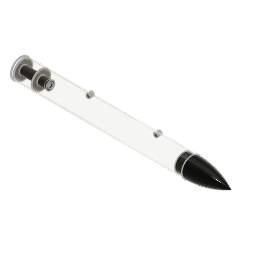
Alpha v1 v2 (Autodesk Fusion 360 design; units mm, degrees)
Autodesk Fusion 360 part; units mm, degrees
sketch "Fuselage" plane through (0, 0, 0) normal (1, 0, 0) x (0, 1, 0)
  circle A0 centre (0, 0) radius 25
  dimension "d1" = 50
  constraint coincident A0.centre origin
  measures "d1" diameter of A0
extrude "Extrude1" add sketch "Fuselage" along normal blind 430 thin wall 2 inside makes body 1
sketch "Ogive" plane through (430, 0, 0) normal (1, 0, 0) x (0, 1, 0)
  circle A0 centre (0, 0) radius 23
  circle A1 centre (0, 0) radius 25
  circle A2 centre (0, 0) radius 25
  line L0 (0, 25) -> (0, -25)
  constraint concentric A0 A2
  constraint coincident A2 L0.start
  constraint coincident A2 L0.end
  constraint vertical L0
extrude "Extrude2" add sketch "Ogive" along normal blind 100 separate body contours A0 L0 | A0 A1 A2 L0 picked at (5.0206, 5.7941) picked at (1.186, 24.2485) makes body 2
sketch "Ogive Curvature Profile" plane through (0, 0, 0) normal (0, -1, 0) x (1, 0, 0)
  line L0 (430, 25) -> (430, -25)
  line L1 (430, -25) -> (530, -25)
  line L2 (530, -25) -> (530, 25)
  line L3 (530, 25) -> (430, 25)
  line L4 (430, 0) -> (430, 25)
  line L5 (430, 0) -> (530, 0)
  circle A0 centre (430, -187.5) radius 212.5
  dimension "d7" = 212.5
  constraint midpoint L0 L4.start
  constraint coincident L0.start L3.end
  constraint midpoint L2 L5.end
  constraint coincident L0.start A0
  measures "d7" distance of L0.start A0.centre
extrude "Extrude3" add sketch "Ogive" along normal blind 100 contours A0 L0 | A0 A1 A2 L0 picked at (-4.3188, 6.3345) picked at (-2.3847, 24.1546) bodies 2
revolve "Revolve1" cut sketch "Ogive Curvature Profile" angle 360 about axis through (430, 0, 0) along (1, 0, 0) contours L0 L4 L5 A0 keep common part bodies 2
sketch "Sholder" plane through (430, 0, 0) normal (-1, 0, 0) x (0, -1, 0)
  circle A0 centre (0, 0) radius 25
  circle A1 centre (0, 0) radius 22.5
  dimension "d11" = 45
  constraint coincident A0.centre A1.centre
  measures "d11" diameter of A1
extrude "Extrude4" add sketch "Sholder" along normal blind 20 contours A1 bodies 2
sketch "Sholder Dent" plane through (410, 0, 0) normal (-1, 0, 0) x (0, -1, 0)
  circle A0 centre (0, 0) radius 22.5
  circle A1 centre (0, 0) radius 17.5
  line L0 (3.75, 17.5) -> (-3.75, 17.5)
  line L1 (-3.75, 17.5) -> (-3.75, -17.5)
  line L2 (-3.75, -17.5) -> (3.75, -17.5)
  line L3 (3.75, -17.5) -> (3.75, 17.5)
  line L4 (3.75, 17.5) -> (-3.75, -17.5) construction
  line L5 (-3.75, 17.5) -> (3.75, -17.5) construction
  dimension "d21" = 35
  dimension "d22" = 7.5
  dimension "d23" = 35
  constraint coincident A0.centre A1.centre
  constraint horizontal L0
  constraint perpendicular L0 L1
  constraint parallel L0 L2
  constraint parallel L1 L3
  constraint coincident L4 A0.centre
  constraint coincident L5 A0.centre
  measures "d21" diameter of A1
  measures "d22" distance of L1.end L2.end
  measures "d23" distance of L0.end L1.end
extrude "Extrude5" cut sketch "Sholder Dent" against normal blind 20 contours A1 L3 | A1 L1 bodies 2
sketch "Sholder Shock Cord hole" plane through (0, 3.75, 0) normal (0, 1, 0) x (-1, 0, 0)
  line L0 (-410, -17.0935) -> (-410, 17.0935)
  line L1 (-410, 17.0935) -> (-430, 17.0935)
  line L2 (-430, 17.0935) -> (-430, -17.0935)
  line L3 (-430, -17.0935) -> (-410, -17.0935)
  circle A0 centre (-420, 0) radius 5
  dimension "d29" = 10
  measures "d29" diameter of A0
extrude "Extrude7" cut sketch "Sholder Shock Cord hole" against normal blind 7.5 contours A0 bodies 2
sketch "Rail Button" plane through (0, 0, 0) normal (0, 0, 1) x (1, 0, 0)
  line L0 (0, 0) -> (5, 0)
  line L1 (0, 0) -> (0, 2)
  line L2 (5, 0) -> (5, 5)
  line L3 (5, 5) -> (1, 5)
  line L4 (1, 5) -> (1, 2)
  line L5 (0, 2) -> (2.1888, 2)
  line L6 (1, 5) -> (1, 8)
  line L7 (0, 8) -> (2.1888, 8)
  line L8 (0, 10) -> (0, 8)
  line L9 (0, 10) -> (5, 10)
  line L10 (5, 10) -> (5, 5)
  dimension "d14" = 5
  dimension "d17" = 2
  dimension "d18" = 5
  dimension "d19" = 4
  constraint horizontal L0
  constraint coincident L0.start L1.start
  constraint perpendicular L0 L1
  constraint perpendicular L0 L2
  constraint perpendicular L2 L3
  constraint parallel L0 L5
  constraint vertical L4
  constraint coincident L4.end L5
  constraint symmetric L0.start L3 L8.start
  constraint symmetric L0.end L3 L9.end
  constraint symmetric L1.end L3 L7.start
  constraint symmetric L2.end L3 L10.end
  constraint symmetric L4.start L3 L6.start
  constraint symmetric L3 L4.end L6.end
  constraint symmetric L3 L5.end L7.end
  measures "d14" distance of L0.start L0.end
  measures "d17" distance of L0.start L1.end
  measures "d18" distance of L0.end L2.end
  measures "d19" distance of L2.end L3.end
revolve "Revolve2" add sketch "Rail Button" angle 360 about axis through (5, 0, 0) along (0, 1, 0) separate body makes body 3
move_body "Move1" bodies 3 to x (1, 0, 0) y (0, 1, 0) z (0, 0, 1) at (-5, -35, 0)
move_body "Move2" bodies 3 to x (1, 0, 0) y (0, 1, 0) z (0, 0, 1) at (315, 60, 0)
extrude "Extrude8" add 1 faces at (313.6899, 25, -1.9935) along direction (0, -1, 0) blind 1.5 on bodies 3 bodies 3
extrude "Extrude9" cut sketch "Fuselage" along normal blind 330 bodies 3
copy_body "CopyPasteBodies1" bodies 3 makes body 4
move_body "Move3" bodies 4 to x (1, 0, 0) y (0, 1, 0) z (0, 0, 1) at (-170, 0, 0)
sketch "Motor" plane through (0, 0, 0) normal (1, 0, 0) x (0, 1, 0)
  circle A0 centre (0, 0) radius 9
  dimension "d36" = 18
  constraint coincident A0.centre origin
  measures "d36" diameter of A0
extrude "Extrude10" add sketch "Motor" along normal blind 70 separate body makes body 5
sketch "Motor Inner Tube" plane through (70, 0, 0) normal (1, 0, 0) x (0, 1, 0)
  circle A0 centre (0, 0) radius 9
  circle A1 centre (0, 0) radius 9.5
  circle A2 centre (0, 0) radius 10.5
  dimension "d39" = 19
  dimension "d40" = 21
  constraint coincident A0.centre A1.centre
  constraint concentric A1 A2
  measures "d39" diameter of A1
  measures "d40" diameter of A2
extrude "Extrude11" add sketch "Motor Inner Tube" along normal blind -70 and the other way blind 0 separate body contours A2 makes body 6
sketch "Motor Retainer" plane through (70, 0, 0) normal (1, 0, 0) x (0, 1, 0)
  circle A0 centre (0, 0) radius 9.5
  circle A1 centre (0, 0) radius 10.5
  circle A2 centre (0, 0) radius 6.5
  dimension "d47" = 13
  constraint concentric A0 A2
  measures "d47" diameter of A2
extrude "Extrude12" add sketch "Motor Retainer" along normal blind 5 contours A0 | A1 bodies 6
sketch "Centering Ring" plane through (0, 0, 0) normal (-1, 0, 0) x (0, -1, 0)
  circle A0 centre (0, 0) radius 9.5
  circle A1 centre (0, 0) radius 10.5
  circle A2 centre (0, 0) radius 23
  dimension "d48" = 46
  constraint coincident A0.centre A1.centre
  measures "d48" diameter of A2
extrude "Extrude13" add sketch "Centering Ring" against normal blind 2 separate body contours A2 makes body 7
move_body "Move5" bodies 7 to x (1, 0, 0) y (0, 1, 0) z (0, 0, 1) at (5, 0, 0)
copy_body "CopyPasteBodies2" bodies 7 makes body 8
move_body "Move4" bodies 8 to x (1, 0, 0) y (0, 1, 0) z (0, 0, 1) at (45, 0, 0)
named bodies: "Fuselage", "Ogive", "Rail Button Front", "Rail Button Back", "Klima Motor D", "Motor Inner Tube", "Centering Ring Back", "Centering Ring", "Centering Ring Front"
